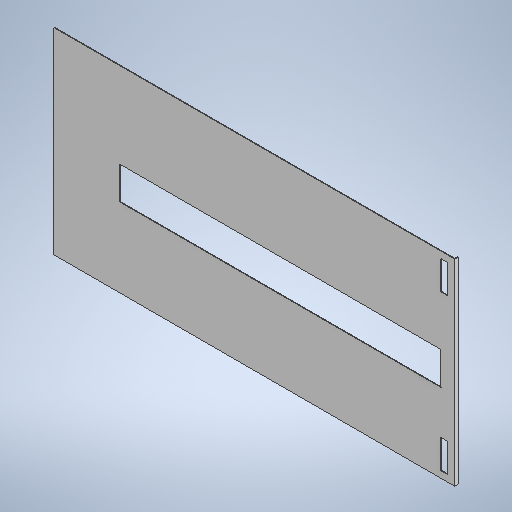
# Autodesk Inventor part: Front Back side
Saved by Autodesk Inventor 2025.1 (Build 291241020, 241B)
## iProperties
Created: 2024-09-24
Part Number: Front Back side
Material: Generic
Document SubType Name: Modeling
Designer: jjk
Density: 1 g/cm^3
Appearance: Default
Author: jjk
Autodesk Inventor part; units mm, degrees
ref_plane "YZ Plane" through (0, 0, 0) normal (1, 0, 0) x (0, 1, 0)
ref_plane "XZ Plane" through (0, 0, 0) normal (0, 1, 0) x (-1, 0, 0)
ref_plane "XY Plane" through (0, 0, 0) normal (0, 0, 1) x (1, 0, 0)
sketch "Sketch1" plane through (0, 0, 0) normal (0, 0, 1) x (1, 0, 0)
  line L0 (0, 0) -> (154.94, 0)
  line L1 (154.94, 0) -> (154.94, 76.2)
  line L2 (154.94, 76.2) -> (0, 76.2)
  line L3 (0, 76.2) -> (0, 0)
  dimension "d0" = 76.2
  dimension "d1" = 154.94
  constraints: 8 end point, 2 parallel, 1 horizontal, 1 perpendicular
  measures "d0" distance of L2.end L0.start
  measures "d1" distance of L0.start L0.end
extrude "Extrusion1" add sketch "Sketch1" along normal blind 0.254
sketch "Sketch2" plane through (0, 0, 0.254) normal (0, 0, 1) x (1, 0, 0)
  line L0 (149.86, 73.66) -> (152.4, 73.66)
  line L1 (152.4, 73.66) -> (152.4, 62.5348)
  line L2 (152.4, 62.5348) -> (149.86, 62.5348)
  line L3 (149.86, 62.5348) -> (149.86, 73.66)
  line L4 (149.86, 13.6652) -> (152.4, 13.6652)
  line L5 (152.4, 13.6652) -> (152.4, 2.54)
  line L6 (152.4, 2.54) -> (149.86, 2.54)
  line L7 (149.86, 2.54) -> (149.86, 13.6652)
  line L8 (154.94, 0) -> (154.94, 76.2) projected
  line L9 (154.94, 76.2) -> (0, 76.2) projected
  line L10 (0, 0) -> (154.94, 0) projected
  point P0 (151.13, 73.66)
  point P1 (151.13, 2.54)
  dimension "d4" = 11.1252
  dimension "d5" = 2.54
  dimension "d6" = 2.54
  dimension "d7" = 2.54
  dimension "d8" = 2.54
  dimension "d9" = 11.1252
  constraints: 16 end point, 4 parallel, 2 horizontal, 2 midpoint, 2 perpendicular, 2 point on line
  measures "d4" distance of L2.end L0.start
  measures "d5" distance of L1.end L2.end
  measures "d6" distance between parallel lines of L8 L1
  measures "d7" distance from line of L9 point (151.13, 73.66)
  measures "d8" distance from line of L10 point (151.13, 2.54)
  measures "d9" distance of L6.end L4.start
extrude "Extrusion2" cut sketch "Sketch2" against normal blind 25.4
sketch "Sketch3" plane through (154.94, 0, 0) normal (1, 0, 0) x (0, 0, -1)
  line L0 (-0.254, 76.2) -> (-0.254, 0) projected
  line L1 (-0.254, 76.2) -> (1.016, 76.2)
  line L2 (1.016, 76.2) -> (1.016, 0)
  line L3 (1.016, 0) -> (-0.254, 0)
  line L4 (-0.254, 0) -> (-0.254, 76.2)
  point P0 (0, 0)
  dimension "d12" = 1.27
  constraints: 8 end point, 2 parallel, 1 horizontal, 1 perpendicular
  measures "d12" distance of L2.end L3.end
extrude "Extrusion3" add sketch "Sketch3" along normal blind 0.254
sketch "Sketch4" plane through (0, 0, 0.254) normal (0, 0, 1) x (1, 0, 0)
  line L0 (149.86, 43.18) -> (25.4, 43.18)
  line L1 (25.4, 43.18) -> (25.4, 30.48)
  line L2 (25.4, 30.48) -> (149.86, 30.48)
  line L3 (149.86, 30.48) -> (149.86, 43.18)
  line L4 (149.86, 62.5348) -> (149.86, 73.66) projected
  line L5 (0, 76.2) -> (155.194, 76.2) projected
  line L6 (0, 76.2) -> (0, 0) projected
  dimension "d15" = 12.7
  dimension "d16" = 0
  dimension "d17" = 33.02
  dimension "d18" = 25.4
  constraints: 8 end point, 2 parallel, 1 horizontal, 1 perpendicular
  measures "d15" distance between parallel lines of L2 L0
  measures "d16" distance between parallel lines of L4 L3
  measures "d17" distance between parallel lines of L5 L0
  measures "d18" distance between parallel lines of L6 L1
extrude "Extrusion4" cut sketch "Sketch4" against normal blind 25.4
body "Solid1"
